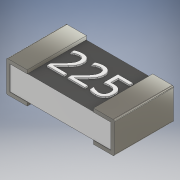
# Autodesk Inventor part: 21-1001
Saved by Autodesk Inventor 2018 (Build 220112000, 112)
## iProperties
Created: 2019-09-21
Part Number: 21-1001
Material: Copper
Document SubType Name: Modeling
Designer: Bradley
Density: 8.94 g/cm^3
Appearance: Smooth - White
Author: Bradley
Autodesk Inventor part; units mm, degrees
ref_plane "YZ Plane" through (0, 0, 0) normal (1, 0, 0) x (0, 1, 0)
ref_plane "XZ Plane" through (0, 0, 0) normal (0, 1, 0) x (-1, 0, 0)
ref_plane "XY Plane" through (0, 0, 0) normal (0, 0, 1) x (1, 0, 0)
sketch "Sketch1" plane through (0, 0, 0) normal (0, 1, 0) x (-1, 0, 0)
  line L0 (0.725, 0.175) -> (-0.725, 0.175)
  line L1 (-0.725, 0.175) -> (-0.725, -0.175)
  line L2 (-0.725, -0.175) -> (0.725, -0.175)
  line L3 (0.725, -0.175) -> (0.725, 0.175)
  line L4 (0.475, 0.175) -> (0.475, 0.225)
  line L5 (0.475, 0.225) -> (0.775, 0.225)
  line L6 (0.775, 0.225) -> (0.775, -0.225)
  line L7 (0.775, -0.225) -> (0.475, -0.225)
  line L8 (0.475, -0.225) -> (0.475, -0.175)
  line L9 (-0.475, 0.175) -> (-0.475, 0.225)
  line L10 (-0.475, 0.225) -> (-0.775, 0.225)
  line L11 (-0.775, 0.225) -> (-0.775, -0.225)
  line L12 (-0.775, -0.225) -> (-0.475, -0.225)
  line L13 (-0.475, -0.175) -> (-0.475, -0.225)
  line L14 (0.475, 0.175) -> (-0.475, 0.175)
  point P0 (0, 0)
  point P1 (0, 0.175)
  point P2 (0.725, 0)
  dimension "d0" = 1.55
  dimension "d1" = 0.05
  dimension "d2" = 0.05
  dimension "d3" = 0.45
  dimension "d4" = 0.3
  constraints: 30 end point, 12 point on line, 7 perpendicular, 3 collinear, 3 midpoint, 2 parallel, 1 horizontal, 1 horizontal alignment, 1 vertical, 1 vertical alignment
  measures "d0" distance between parallel lines of L11 L6
  measures "d1" distance of L7.end L8.end
  measures "d2" distance between parallel lines of L6 L3
  measures "d3" distance of L5.end L6.end
  measures "d4" distance of L6.end L7.end
extrude "Extrusion1" add sketch "Sketch1" along normal mid plane 0.85 contours L0 L4 L5 L6 L7 L8 L2 L3 | L0 L1 L2 L13 L12 L11 L10 L9
extrude "Extrusion2" add sketch "Sketch1" along normal mid plane 0.84 contours L3 L2 L1 L0
sketch "Sketch2" plane through (-0.475, -0.42, 0.175) normal (0, 0, 1) x (1, 0, 0)
  line L0 (0, 0) -> (0, 0.84) projected
  line L1 (0.95, 0) -> (0, 0) projected
  line L2 (0.95, 0) -> (0.95, 0.84) projected
  line L3 (0, 0.84) -> (0.95, 0.84) projected
  line L4 (0, 0.42) -> (0.95, 0.42) construction
  line L5 (0.3006, 0.22) -> (0.0539, 0.22)
  line L6 (0.0539, 0.22) -> (0.0539, 0.2767)
  spline S0 degree 2 poles (0.0539, 0.2767) (0.0805, 0.3017) (0.1278, 0.348) (0.1505, 0.373) knots 0 0 0 1 2 2 2
  spline S1 degree 2 poles (0.1505, 0.373) (0.1962, 0.4232) (0.2296, 0.4835) (0.2296, 0.5156) knots 0 0 0 1 2 2 2
  spline S2 degree 2 poles (0.2296, 0.5156) (0.2296, 0.5325) (0.2192, 0.5578) (0.2098, 0.5659) knots 0 0 0 1 2 2 2
  spline S3 degree 2 poles (0.2098, 0.5659) (0.2004, 0.574) (0.1758, 0.5821) (0.1609, 0.5821) knots 0 0 0 1 2 2 2
  spline S4 degree 2 poles (0.1609, 0.5821) (0.1466, 0.5821) (0.1175, 0.5749) (0.1042, 0.5694) knots 0 0 0 1 2 2 2
  spline S5 degree 2 poles (0.1042, 0.5694) (0.0928, 0.5649) (0.0718, 0.5519) (0.0653, 0.5474) knots 0 0 0 1 2 2 2
  line L7 (0.0653, 0.5474) -> (0.0624, 0.5474)
  line L8 (0.0624, 0.5474) -> (0.0624, 0.6044)
  spline S6 degree 2 poles (0.0624, 0.6044) (0.0789, 0.6125) (0.1382, 0.6284) (0.1648, 0.6284) knots 0 0 0 1 2 2 2
  spline S7 degree 2 poles (0.1648, 0.6284) (0.2209, 0.6284) (0.2841, 0.5691) (0.2841, 0.5185) knots 0 0 0 1 2 2 2
  spline S8 degree 2 poles (0.2841, 0.5185) (0.2841, 0.4949) (0.2731, 0.4553) (0.2633, 0.4385) knots 0 0 0 1 2 2 2
  spline S9 degree 2 poles (0.2633, 0.4385) (0.2536, 0.421) (0.2254, 0.3866) (0.2098, 0.3701) knots 0 0 0 1 2 2 2
  spline S10 degree 2 poles (0.2098, 0.3701) (0.1846, 0.3425) (0.1226, 0.2835) (0.1042, 0.2664) knots 0 0 0 1 2 2 2
  line L9 (0.1042, 0.2664) -> (0.3006, 0.2664)
  line L10 (0.3006, 0.2664) -> (0.3006, 0.22)
  line L11 (0.6008, 0.22) -> (0.3541, 0.22)
  line L12 (0.3541, 0.22) -> (0.3541, 0.2767)
  spline S11 degree 2 poles (0.3541, 0.2767) (0.3807, 0.3017) (0.428, 0.348) (0.4507, 0.373) knots 0 0 0 1 2 2 2
  spline S12 degree 2 poles (0.4507, 0.373) (0.4964, 0.4232) (0.5298, 0.4835) (0.5298, 0.5156) knots 0 0 0 1 2 2 2
  spline S13 degree 2 poles (0.5298, 0.5156) (0.5298, 0.5325) (0.5194, 0.5578) (0.51, 0.5659) knots 0 0 0 1 2 2 2
  spline S14 degree 2 poles (0.51, 0.5659) (0.5006, 0.574) (0.476, 0.5821) (0.4611, 0.5821) knots 0 0 0 1 2 2 2
  spline S15 degree 2 poles (0.4611, 0.5821) (0.4468, 0.5821) (0.4176, 0.5749) (0.4043, 0.5694) knots 0 0 0 1 2 2 2
  spline S16 degree 2 poles (0.4043, 0.5694) (0.393, 0.5649) (0.3719, 0.5519) (0.3654, 0.5474) knots 0 0 0 1 2 2 2
  line L13 (0.3654, 0.5474) -> (0.3625, 0.5474)
  line L14 (0.3625, 0.5474) -> (0.3625, 0.6044)
  spline S17 degree 2 poles (0.3625, 0.6044) (0.3791, 0.6125) (0.4384, 0.6284) (0.465, 0.6284) knots 0 0 0 1 2 2 2
  spline S18 degree 2 poles (0.465, 0.6284) (0.521, 0.6284) (0.5842, 0.5691) (0.5842, 0.5185) knots 0 0 0 1 2 2 2
  spline S19 degree 2 poles (0.5842, 0.5185) (0.5842, 0.4949) (0.5732, 0.4553) (0.5635, 0.4385) knots 0 0 0 1 2 2 2
  spline S20 degree 2 poles (0.5635, 0.4385) (0.5538, 0.421) (0.5256, 0.3866) (0.51, 0.3701) knots 0 0 0 1 2 2 2
  spline S21 degree 2 poles (0.51, 0.3701) (0.4847, 0.3425) (0.4228, 0.2835) (0.4043, 0.2664) knots 0 0 0 1 2 2 2
  line L15 (0.4043, 0.2664) -> (0.6008, 0.2664)
  line L16 (0.6008, 0.2664) -> (0.6008, 0.22)
  spline S22 degree 2 poles (0.8967, 0.3471) (0.8967, 0.3182) (0.8782, 0.2689) (0.8614, 0.2508) knots 0 0 0 1 2 2 2
  spline S23 degree 2 poles (0.8614, 0.2508) (0.8445, 0.2326) (0.7943, 0.2116) (0.7632, 0.2116) knots 0 0 0 1 2 2 2
  spline S24 degree 2 poles (0.7632, 0.2116) (0.7346, 0.2116) (0.6789, 0.2242) (0.6585, 0.2343) knots 0 0 0 1 2 2 2
  line L17 (0.6585, 0.2343) -> (0.6585, 0.291)
  line L18 (0.6585, 0.291) -> (0.6624, 0.291)
  spline S25 degree 2 poles (0.6624, 0.291) (0.6685, 0.2865) (0.6915, 0.2748) (0.7055, 0.2696) knots 0 0 0 1 2 2 2
  spline S26 degree 2 poles (0.7055, 0.2696) (0.7214, 0.2641) (0.7476, 0.2579) (0.7641, 0.2579) knots 0 0 0 1 2 2 2
  spline S27 degree 2 poles (0.7641, 0.2579) (0.7803, 0.2579) (0.8108, 0.2696) (0.8218, 0.2822) knots 0 0 0 1 2 2 2
  spline S28 degree 2 poles (0.8218, 0.2822) (0.8319, 0.2942) (0.8423, 0.326) (0.8423, 0.3474) knots 0 0 0 1 2 2 2
  spline S29 degree 2 poles (0.8423, 0.3474) (0.8423, 0.3688) (0.8306, 0.396) (0.8196, 0.4051) knots 0 0 0 1 2 2 2
  spline S30 degree 2 poles (0.8196, 0.4051) (0.8082, 0.4151) (0.7745, 0.4236) (0.7541, 0.4236) knots 0 0 0 1 2 2 2
  spline S31 degree 2 poles (0.7541, 0.4236) (0.7321, 0.4236) (0.6883, 0.4168) (0.675, 0.4138) knots 0 0 0 1 2 2 2
  line L19 (0.675, 0.4138) -> (0.675, 0.62)
  line L20 (0.675, 0.62) -> (0.8944, 0.62)
  line L21 (0.8944, 0.62) -> (0.8944, 0.573)
  line L22 (0.8944, 0.573) -> (0.7265, 0.573)
  line L23 (0.7265, 0.573) -> (0.7265, 0.4664)
  spline S32 degree 2 poles (0.7265, 0.4664) (0.7363, 0.4676) (0.7551, 0.4686) (0.7628, 0.4686) knots 0 0 0 1 2 2 2
  spline S33 degree 2 poles (0.7628, 0.4686) (0.7936, 0.4686) (0.8361, 0.4586) (0.8556, 0.4437) knots 0 0 0 1 2 2 2
  spline S34 degree 2 poles (0.8556, 0.4437) (0.8753, 0.4288) (0.8967, 0.3834) (0.8967, 0.3471) knots 0 0 0 1 2 2 2
  point P0 (0.475, 0.42)
  constraints: 2 end point, 2 midpoint, 1 horizontal
extrude "Extrusion3" add sketch "Sketch2" along normal blind 0.02 contours L5 L6 S0 S1 S2 S3 S4 S5 L7 L8 S6 S7 S8 S9 S10 L9 L10 | L11 L12 S11 S12 S13 S14 S15 S16 L13 L14 S17 S18 S19 S20 S21 L15 L16 | S22 S23 S24 L17 L18 S25 S26 S27 S28 S29 S30 S31 L19 L20 L21 L22 L23 S32 S33 S34
fillet "Fillet1" radius 0.02 4 edges at (-0.775, 0, 0.225) (-0.775, 0, -0.225) (0.775, 0, 0.225) (0.775, 0, -0.225)
equation "\"d2\" = d1"
body "Solid1"
